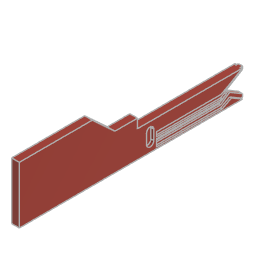
3ks (Autodesk Fusion 360 design; units mm, degrees)
Autodesk Fusion 360 part; units mm, degrees
note: some values were not read from the file. Set by a fixed rule: which face or edge a step refers to.
sketch "blade" plane through (0, 0, 0) normal (1, 0, 0) x (0, 1, 0)
  line L0 (0, 0) -> (0, 0.75) construction
  line L1 (0, 0.75) -> (25.25, 0.75)
  line L2 (25.25, 0.75) -> (25.25, 8.75)
  line L3 (25.25, 8.75) -> (0, 8.75)
  line L4 (0, 8.75) -> (0, 0.75)
  dimension "d14" = 0.75
  dimension "d15" = 25.25
  dimension "d16" = 8
  constraint coincident L0.start origin
  constraint vertical L0
  constraint horizontal L1
  constraint vertical L2
  constraint horizontal L3
  constraint vertical L4
  measures "d14" distance of L0.start L0.end
  measures "d15" distance of L0.end L1.end
  measures "d16" distance of L0.end L3.end
extrude "Extrude1" add sketch "blade" along normal blind 1.1 makes body 1
sketch "single track" plane through (1.1, 0, 0) normal (1, 0, 0) x (0, 1, 0)
  line L0 (0, 8.75) -> (0, 0.75)
  line L1 (0, 0.75) -> (25.25, 0.75)
  line L2 (25.25, 0.75) -> (25.25, 8.75)
  line L3 (25.25, 8.75) -> (0, 8.75)
  line L4 (0, 0.75) -> (0.9, 0.75) construction
  line L5 (0.9, 0.75) -> (4.4, 0.75) construction
  line L6 (4.4, 0.75) -> (7.9, 0.75) construction
  line L7 (7.9, 0.75) -> (11.4, 0.75) construction
  line L8 (11.4, 0.75) -> (14.9, 0.75) construction
  line L9 (14.9, 0.75) -> (18.4, 0.75) construction
  line L10 (0.9, 0.75) -> (0.9, 2.75) construction
  line L11 (4.4, 0.75) -> (4.4, 2.75) construction
  line L12 (7.9, 0.75) -> (7.9, 2.75) construction
  line L13 (11.4, 0.75) -> (11.4, 2.75) construction
  line L14 (14.9, 0.75) -> (14.9, 2.75) construction
  line L15 (18.4, 0.75) -> (18.4, 2.75) construction
  circle A0 centre (0.9, 2.75) radius 0.6375 construction
  circle A1 centre (4.4, 2.75) radius 0.6375 construction
  circle A2 centre (7.9, 2.75) radius 0.6375 construction
  circle A3 centre (11.4, 2.75) radius 0.6375 construction
  circle A4 centre (14.9, 2.75) radius 0.6375 construction
  circle A5 centre (18.4, 2.75) radius 0.6375 construction
  line L16 (0.9, 2.75) -> (0, 2.75)
  line L17 (0, 0.75) -> (0, 2.75) construction
  line L18 (0.9, 2.75) -> (1.2375, 2.75)
  line L19 (4.4, 2.75) -> (4.0625, 2.75)
  line L20 (4.4, 2.75) -> (4.7375, 2.75)
  line L21 (7.9, 2.75) -> (7.5625, 2.75)
  line L22 (7.9, 2.75) -> (8.2375, 2.75)
  line L23 (11.4, 2.75) -> (11.0625, 2.75)
  line L24 (11.4, 2.75) -> (11.7375, 2.75)
  line L25 (14.9, 2.75) -> (14.5625, 2.75)
  line L26 (14.9, 2.75) -> (15.2375, 2.75)
  line L27 (18.4, 2.75) -> (18.0625, 2.75)
  line L28 (18.4, 0.75) -> (21.9, 0.75) construction
  line L29 (18.4, 2.75) -> (18.7375, 2.75)
  line L30 (21.9, 0.75) -> (21.9, 4.75) construction
  line L31 (21.9, 4.75) -> (25.25, 4.75)
  line L32 (21.9, 4.75) -> (21.5625, 4.75)
  line L33 (1.2375, 2.75) -> (4.0625, 2.75)
  line L34 (4.7375, 2.75) -> (7.5625, 2.75)
  line L35 (8.2375, 2.75) -> (11.0625, 2.75)
  line L36 (11.7375, 2.75) -> (14.5625, 2.75)
  line L37 (15.2375, 2.75) -> (18.0625, 2.75)
  line L38 (18.7375, 2.75) -> (21.5625, 4.75)
  dimension "d19" = 0.9
  dimension "d20" = 3.5
  dimension "d21" = 3.5
  dimension "d22" = 3.5
  dimension "d23" = 3.5
  dimension "d24" = 3.5
  dimension "d25" = 2
  dimension "d26" = 2
  dimension "d27" = 2
  dimension "d28" = 2
  dimension "d29" = 2
  dimension "d30" = 2
  dimension "d31" = 1.275
  dimension "d32" = 1.275
  dimension "d33" = 1.275
  dimension "d34" = 1.275
  dimension "d35" = 1.275
  dimension "d36" = 1.275
  dimension "d37" = 0.3375
  dimension "d38" = 0.3375
  dimension "d39" = 0.3375
  dimension "d40" = 0.3375
  dimension "d41" = 0.3375
  dimension "d42" = 0.3375
  dimension "d43" = 0.3375
  dimension "d44" = 0.3375
  dimension "d45" = 0.3375
  dimension "d46" = 0.3375
  dimension "d47" = 3.5
  dimension "d48" = 0.3375
  dimension "d49" = 0.3375
  constraint coincident L0.end L1.start
  constraint perpendicular L0 L4
  constraint parallel L1 L5
  constraint parallel L1 L6
  constraint parallel L1 L7
  constraint parallel L1 L8
  constraint parallel L1 L9
  constraint perpendicular L5 L10
  constraint perpendicular L5 L11
  constraint perpendicular L7 L12
  constraint perpendicular L8 L13
  constraint perpendicular L1 L14
  constraint perpendicular L9 L15
  constraint coincident L10.end A0.centre
  constraint coincident L11.end A1.centre
  constraint coincident L12.end A2.centre
  constraint coincident L13.end A3.centre
  constraint coincident L14.end A4.centre
  constraint coincident L15.end A5.centre
  constraint coincident L0 L16.end
  constraint perpendicular L0 L16
  constraint perpendicular L10 L18
  constraint perpendicular L11 L19
  constraint perpendicular L11 L20
  constraint perpendicular L12 L21
  constraint perpendicular L12 L22
  constraint perpendicular L13 L23
  constraint perpendicular L13 L24
  constraint perpendicular L14 L25
  constraint perpendicular L14 L26
  constraint perpendicular L15 L27
  constraint perpendicular L15 L28
  constraint perpendicular L15 L29
  constraint perpendicular L28 L30
  constraint midpoint L2 L31.end
  constraint perpendicular L2 L31
  constraint perpendicular L30 L32
  measures "d19" distance of L0.end L4.end
  measures "d20" distance of L4.end L5.end
  measures "d21" distance of L5.end L6.end
  measures "d22" distance of L6.end L7.end
  measures "d23" distance of L7.end L8.end
  measures "d24" distance of L8.end L9.end
  measures "d25" distance of L4.end L10.end
  measures "d26" distance of L5.end L11.end
  measures "d27" distance of L6.end L12.end
  measures "d28" distance of L7.end L13.end
  measures "d29" distance of L8.end L14.end
  measures "d30" distance of L9.end L15.end
  measures "d31" diameter of A0
  measures "d32" diameter of A1
  measures "d33" diameter of A2
  measures "d34" diameter of A3
  measures "d35" diameter of A4
  measures "d36" diameter of A5
  measures "d37" distance of L10.end L18.end
  measures "d38" distance of L11.end L19.end
  measures "d39" distance of L11.end L20.end
  measures "d40" distance of L12.end L21.end
  measures "d41" distance of L12.end L22.end
  measures "d42" distance of L13.end L23.end
  measures "d43" distance of L13.end L24.end
  measures "d44" distance of L14.end L25.end
  measures "d45" distance of L14.end L26.end
  measures "d46" distance of L15.end L27.end
  measures "d47" distance of L9.end L28.end
  measures "d48" distance of L15.end L29.end
  measures "d49" distance of L30.end L32.end
sketch "single track cutter" plane through (0, 0, 0) normal (0, -1, 0) x (1, 0, 0)
  line L0 (0, 0.75) -> (1.1, 0.75)
  line L1 (1.1, 0.75) -> (1.1, 8.75)
  line L2 (1.1, 8.75) -> (0, 8.75)
  line L3 (0, 8.75) -> (0, 0.75)
  line L4 (1.1, 2.75) -> (1.1, 2.1125)
  line L5 (1.1, 2.75) -> (1.1, 3.3875)
  line L6 (1.1, 3.3875) -> (0.1, 3.3875)
  line L7 (0.1, 3.3875) -> (0.1, 2.1125)
  line L8 (0.1, 2.1125) -> (1.1, 2.1125)
  point P0 (1.1, 2.75)
  dimension "d50" = 0.6375
  dimension "d51" = 0.6375
  dimension "d52" = 1
  constraint vertical L4
  constraint coincident P0 L4.start
  constraint parallel L1 L5
  constraint perpendicular L5 L6
  constraint perpendicular L6 L7
  constraint perpendicular L4 L8
  measures "d50" distance of P0 L4.end
  measures "d51" distance of P0 L5.end
  measures "d52" distance of L5.end L6.end
sketch "double track" plane through (1.1, 0, 0) normal (1, 0, 0) x (0, 1, 0)
  line L0 (0, 8.75) -> (0, 0.75)
  line L1 (0, 0.75) -> (25.25, 0.75)
  line L2 (25.25, 0.75) -> (25.25, 8.75)
  line L3 (25.25, 8.75) -> (0, 8.75)
  line L4 (0, 0.75) -> (0.9, 0.75) construction
  line L5 (0.9, 0.75) -> (4.4, 0.75) construction
  line L6 (4.4, 0.75) -> (7.9, 0.75) construction
  line L7 (7.9, 0.75) -> (11.4, 0.75) construction
  line L8 (11.4, 0.75) -> (14.9, 0.75) construction
  line L9 (14.9, 0.75) -> (18.4, 0.75) construction
  line L10 (18.4, 0.75) -> (21.9, 0.75) construction
  line L11 (21.9, 0.75) -> (21.9, 4.75) construction
  line L12 (21.9, 4.75) -> (25.25, 4.75) construction
  line L13 (0.9, 0.75) -> (0.9, 3.25) construction
  line L14 (4.4, 0.75) -> (4.4, 3.25) construction
  line L15 (7.9, 0.75) -> (7.9, 3.25) construction
  line L16 (11.4, 0.75) -> (11.4, 3.25) construction
  line L17 (14.9, 0.75) -> (14.9, 3.25) construction
  line L18 (18.4, 0.75) -> (18.4, 3.25) construction
  line L19 (0.9, 3.25) -> (0.9, 2) construction
  line L20 (0.9, 3.25) -> (0.9, 4.5) construction
  line L21 (4.4, 3.25) -> (4.4, 2) construction
  line L22 (4.4, 3.25) -> (4.4, 4.5) construction
  line L23 (7.9, 3.25) -> (7.9, 2) construction
  line L24 (7.9, 3.25) -> (7.9, 4.5) construction
  line L25 (11.4, 3.25) -> (11.4, 2) construction
  line L26 (11.4, 3.25) -> (11.4, 4.5) construction
  line L27 (14.9, 3.25) -> (14.9, 2) construction
  line L28 (14.9, 3.25) -> (14.9, 4.5) construction
  line L29 (18.4, 3.25) -> (18.4, 2) construction
  line L30 (18.4, 3.25) -> (18.4, 4.5) construction
  line L31 (21.9, 4.75) -> (21.9, 3.5) construction
  line L32 (21.9, 4.75) -> (21.9, 6) construction
  circle A0 centre (0.9, 2) radius 0.6375 construction
  circle A1 centre (0.9, 4.5) radius 0.6375 construction
  circle A2 centre (4.4, 2) radius 0.6375 construction
  circle A3 centre (4.4, 4.5) radius 0.6375 construction
  circle A4 centre (7.9, 2) radius 0.6375 construction
  circle A5 centre (7.9, 4.5) radius 0.6375 construction
  circle A6 centre (11.4, 2) radius 0.6375 construction
  circle A7 centre (11.4, 4.5) radius 0.6375 construction
  circle A8 centre (14.9, 2) radius 0.6375 construction
  circle A9 centre (14.9, 4.5) radius 0.6375 construction
  circle A10 centre (18.4, 2) radius 0.6375 construction
  circle A11 centre (18.4, 4.5) radius 0.6375 construction
  line L33 (0.9, 2) -> (0, 2)
  line L34 (0.9, 4.5) -> (0, 4.5)
  line L35 (0, 0.75) -> (0, 2) construction
  line L36 (0, 0.75) -> (0, 4.5) construction
  line L37 (0.9, 2) -> (1.2375, 2)
  line L38 (4.4, 2) -> (4.0625, 2)
  line L39 (4.4, 2) -> (4.7375, 2)
  line L40 (7.9, 2) -> (7.5625, 2)
  line L41 (7.9, 2) -> (8.2375, 2)
  line L42 (11.4, 2) -> (11.0625, 2)
  line L43 (11.4, 2) -> (11.7375, 2)
  line L44 (14.9, 2) -> (14.5625, 2)
  line L45 (14.9, 2) -> (15.2375, 2)
  line L46 (18.4, 2) -> (18.0625, 2)
  line L47 (18.4, 2) -> (18.7375, 2)
  line L48 (21.9, 3.5) -> (21.5625, 3.5) construction
  line L49 (0.9, 4.5) -> (1.2375, 4.5)
  line L50 (4.4, 4.5) -> (4.0625, 4.5)
  line L51 (4.4, 4.5) -> (4.7375, 4.5)
  line L52 (7.9, 4.5) -> (7.5625, 4.5)
  line L53 (7.9, 4.5) -> (8.2375, 4.5)
  line L54 (11.4, 4.5) -> (11.0625, 4.5)
  line L55 (11.4, 4.5) -> (11.7375, 4.5)
  line L56 (14.9, 4.5) -> (14.5625, 4.5)
  line L57 (14.9, 4.5) -> (15.2375, 4.5)
  line L58 (18.4, 4.5) -> (18.0625, 4.5)
  line L59 (18.4, 4.5) -> (18.7375, 4.5)
  line L60 (21.9, 6) -> (21.5625, 6) construction
  line L61 (1.2375, 2) -> (4.0625, 2)
  line L62 (4.7375, 2) -> (7.5625, 2)
  line L63 (8.2375, 2) -> (11.0625, 2)
  line L64 (11.7375, 2) -> (14.5625, 2)
  line L65 (15.2375, 2) -> (18.0625, 2)
  line L66 (18.7375, 2) -> (21.5625, 3.5)
  line L67 (21.5625, 3.5) -> (25.25, 1.3192)
  line L68 (21.5625, 3.5) -> (25.25, 3.5) construction
  line L69 (25.25, 1.3192) -> (26.3259, 0.6829)
  line L70 (1.2375, 4.5) -> (4.0625, 4.5)
  line L71 (4.7375, 4.5) -> (7.5625, 4.5)
  line L72 (8.2375, 4.5) -> (11.0625, 4.5)
  line L73 (11.7375, 4.5) -> (14.5625, 4.5)
  line L74 (15.2375, 4.5) -> (18.0625, 4.5)
  line L75 (18.7375, 4.5) -> (21.5625, 6)
  line L76 (21.5625, 6) -> (25.25, 8.1808)
  line L77 (21.5625, 6) -> (25.25, 6) construction
  line L78 (25.25, 8.1808) -> (26.3259, 8.8171)
  dimension "d53" = 0.9
  dimension "d54" = 3.5
  dimension "d55" = 3.5
  dimension "d56" = 3.5
  dimension "d57" = 3.5
  dimension "d58" = 3.5
  dimension "d59" = 3.5
  dimension "d60" = 2.5
  dimension "d61" = 2.5
  dimension "d62" = 2.5
  dimension "d63" = 2.5
  dimension "d64" = 2.5
  dimension "d65" = 2.5
  dimension "d66" = 1.25
  dimension "d67" = 1.25
  dimension "d68" = 1.25
  dimension "d69" = 1.25
  dimension "d70" = 1.25
  dimension "d71" = 1.25
  dimension "d72" = 1.25
  dimension "d73" = 1.25
  dimension "d74" = 1.25
  dimension "d75" = 1.25
  dimension "d76" = 1.25
  dimension "d77" = 1.25
  dimension "d78" = 1.25
  dimension "d79" = 1.25
  dimension "d80" = 1.275
  dimension "d81" = 1.275
  dimension "d82" = 1.275
  dimension "d83" = 1.275
  dimension "d84" = 1.275
  dimension "d85" = 1.275
  dimension "d86" = 1.275
  dimension "d87" = 1.275
  dimension "d88" = 1.275
  dimension "d89" = 1.275
  dimension "d90" = 1.275
  dimension "d91" = 1.275
  dimension "d92" = 0.3375
  dimension "d93" = 0.3375
  dimension "d94" = 0.3375
  dimension "d95" = 0.3375
  dimension "d96" = 0.3375
  dimension "d97" = 0.3375
  dimension "d98" = 0.3375
  dimension "d99" = 0.3375
  dimension "d100" = 0.3375
  dimension "d101" = 0.3375
  dimension "d102" = 0.3375
  dimension "d103" = 0.3375
  dimension "d104" = 0.3375
  dimension "d105" = 0.3375
  dimension "d106" = 0.3375
  dimension "d107" = 0.3375
  dimension "d108" = 0.3375
  dimension "d109" = 0.3375
  dimension "d110" = 0.3375
  dimension "d111" = 0.3375
  dimension "d112" = 0.3375
  dimension "d113" = 0.3375
  dimension "d114" = 0.3375
  dimension "d115" = 0.3375
  dimension "d116" = 149.4
  dimension "d117" = 1.25
  dimension "d118" = 149.4
  dimension "d119" = 1.25
  constraint coincident L0.end L1.start
  constraint perpendicular L0 L4
  constraint parallel L1 L5
  constraint parallel L1 L6
  constraint parallel L1 L7
  constraint parallel L1 L8
  constraint parallel L1 L9
  constraint parallel L1 L10
  constraint perpendicular L10 L11
  constraint midpoint L2 L12.end
  constraint perpendicular L2 L12
  constraint perpendicular L5 L13
  constraint perpendicular L5 L14
  constraint perpendicular L7 L15
  constraint perpendicular L1 L16
  constraint perpendicular L8 L17
  constraint perpendicular L9 L18
  constraint parallel L13 L19
  constraint parallel L19 L20
  constraint parallel L14 L21
  constraint parallel L21 L22
  constraint parallel L15 L23
  constraint parallel L15 L24
  constraint parallel L16 L25
  constraint parallel L25 L26
  constraint parallel L17 L27
  constraint parallel L17 L28
  constraint parallel L18 L29
  constraint parallel L18 L30
  constraint perpendicular L12 L31
  constraint perpendicular L12 L32
  constraint coincident L19.end A0.centre
  constraint coincident L20.end A1.centre
  constraint coincident L21.end A2.centre
  constraint coincident L22.end A3.centre
  constraint coincident L23.end A4.centre
  constraint coincident L24.end A5.centre
  constraint coincident L25.end A6.centre
  constraint coincident L26.end A7.centre
  constraint coincident L27.end A8.centre
  constraint coincident L28.end A9.centre
  constraint coincident L29.end A10.centre
  constraint coincident L30.end A11.centre
  constraint coincident L0 L33.end
  constraint perpendicular L0 L33
  constraint coincident L0 L34.end
  constraint perpendicular L0 L34
  constraint perpendicular L13 L37
  constraint perpendicular L14 L38
  constraint perpendicular L21 L39
  constraint perpendicular L15 L40
  constraint perpendicular L15 L41
  constraint perpendicular L16 L42
  constraint perpendicular L16 L43
  constraint perpendicular L17 L44
  constraint perpendicular L17 L45
  constraint perpendicular L29 L46
  constraint perpendicular L29 L47
  constraint perpendicular L31 L48
  constraint perpendicular L20 L49
  constraint perpendicular L22 L50
  constraint perpendicular L22 L51
  constraint perpendicular L24 L52
  constraint perpendicular L24 L53
  constraint perpendicular L26 L54
  constraint perpendicular L26 L55
  constraint perpendicular L28 L56
  constraint perpendicular L28 L57
  constraint perpendicular L30 L58
  constraint perpendicular L30 L59
  constraint perpendicular L32 L60
  constraint horizontal L68
  constraint coincident L2 L67.end
  constraint coincident L2 L68.end
  constraint parallel L67 L69
  constraint horizontal L77
  constraint coincident L2 L76.end
  constraint coincident L2 L77.end
  constraint parallel L76 L78
  measures "d53" distance of L0.end L4.end
  measures "d54" distance of L4.end L5.end
  measures "d55" distance of L5.end L6.end
  measures "d56" distance of L6.end L7.end
  measures "d57" distance of L7.end L8.end
  measures "d58" distance of L8.end L9.end
  measures "d59" distance of L9.end L10.end
  measures "d60" distance of L4.end L13.end
  measures "d61" distance of L5.end L14.end
  measures "d62" distance of L6.end L15.end
  measures "d63" distance of L7.end L16.end
  measures "d64" distance of L8.end L17.end
  measures "d65" distance of L9.end L18.end
  measures "d66" distance of L13.end L19.end
  measures "d67" distance of L13.end L20.end
  measures "d68" distance of L14.end L21.end
  measures "d69" distance of L14.end L22.end
  measures "d70" distance of L15.end L23.end
  measures "d71" distance of L15.end L24.end
  measures "d72" distance of L16.end L25.end
  measures "d73" distance of L16.end L26.end
  measures "d74" distance of L17.end L27.end
  measures "d75" distance of L17.end L28.end
  measures "d76" distance of L18.end L29.end
  measures "d77" distance of L18.end L30.end
  measures "d78" distance of L11.end L31.end
  measures "d79" distance of L11.end L32.end
  measures "d80" diameter of A0
  measures "d81" diameter of A1
  measures "d82" diameter of A2
  measures "d83" diameter of A3
  measures "d84" diameter of A4
  measures "d85" diameter of A5
  measures "d86" diameter of A6
  measures "d87" diameter of A7
  measures "d88" diameter of A8
  measures "d89" diameter of A9
  measures "d90" diameter of A10
  measures "d91" diameter of A11
  measures "d92" distance of L19.end L37.end
  measures "d93" distance of L21.end L38.end
  measures "d94" distance of L21.end L39.end
  measures "d95" distance of L23.end L40.end
  measures "d96" distance of L23.end L41.end
  measures "d97" distance of L25.end L42.end
  measures "d98" distance of L25.end L43.end
  measures "d99" distance of L27.end L44.end
  measures "d100" distance of L27.end L45.end
  measures "d101" distance of L29.end L46.end
  measures "d102" distance of L29.end L47.end
  measures "d103" distance of L31.end L48.end
  measures "d104" distance of L20.end L49.end
  measures "d105" distance of L22.end L50.end
  measures "d106" distance of L22.end L51.end
  measures "d107" distance of L24.end L52.end
  measures "d108" distance of L24.end L53.end
  measures "d109" distance of L26.end L54.end
  measures "d110" distance of L26.end L55.end
  measures "d111" distance of L28.end L56.end
  measures "d112" distance of L28.end L57.end
  measures "d113" distance of L30.end L58.end
  measures "d114" distance of L30.end L59.end
  measures "d115" distance of L32.end L60.end
  measures "d116" angle of L67 L68
  measures "d117" distance of L67.end L69.end
  measures "d118" angle of L76 L77
  measures "d119" distance of L76.end L78.end
sketch "double track cutter" plane through (0, 0, 0) normal (0, -1, 0) x (1, 0, 0)
  line L0 (0, 0.75) -> (1.1, 0.75)
  line L1 (1.1, 0.75) -> (1.1, 8.75)
  line L2 (1.1, 8.75) -> (0, 8.75)
  line L3 (0, 8.75) -> (0, 0.75)
  line L4 (1.1, 2) -> (1.1, 1.3625)
  line L5 (1.1, 4.5) -> (1.1, 3.8625)
  line L6 (1.1, 2) -> (1.1, 2.6375)
  line L7 (1.1, 4.5) -> (1.1, 5.1375)
  line L8 (1.1, 1.3625) -> (0.6, 1.3625)
  line L9 (1.1, 3.8625) -> (0.6, 3.8625)
  line L10 (0.6, 1.3625) -> (0.6, 2.6375)
  line L11 (0.6, 2.6375) -> (1.1, 2.6375)
  line L12 (0.6, 3.8625) -> (0.6, 5.1375)
  line L13 (0.6, 5.1375) -> (1.1, 5.1375)
  point P0 (1.1, 2)
  point P1 (1.1, 4.5)
  dimension "d120" = 0.6375
  dimension "d121" = 0.6375
  dimension "d122" = 0.6375
  dimension "d123" = 0.6375
  dimension "d124" = 0.5
  dimension "d125" = 0.5
  constraint vertical L4
  constraint coincident P0 L4.start
  constraint vertical L5
  constraint coincident P1 L5.start
  constraint parallel L1 L6
  constraint parallel L1 L7
  constraint perpendicular L4 L8
  constraint perpendicular L5 L9
  constraint perpendicular L8 L10
  constraint perpendicular L6 L11
  constraint perpendicular L9 L12
  constraint perpendicular L7 L13
  measures "d120" distance of P0 L4.end
  measures "d121" distance of P1 L5.end
  measures "d122" distance of P0 L6.end
  measures "d123" distance of P1 L7.end
  measures "d124" distance of L4.end L8.end
  measures "d125" distance of L5.end L9.end
extrude "sidebar hole extension" add 1 faces at (0.3667, 0, 6.0833) along direction (0, -1, 0) blind 5.5 on bodies 1 bodies 1
sketch "sidebar hole" plane through (1.1, 0, 0) normal (1, 0, 0) x (0, 1, 0)
  line L0 (-5.5, 0.75) -> (25.25, 0.75)
  line L1 (25.25, 0.75) -> (25.25, 8.75)
  line L2 (25.25, 8.75) -> (-5.5, 8.75)
  line L3 (-5.5, 8.75) -> (-5.5, 0.75)
  line L4 (-5.5, 0.75) -> (0, 0.75) construction
  line L5 (0, 0.75) -> (0, 4.75) construction
  line L6 (0, 4.75) -> (-2.9, 4.75) construction
  line L7 (-2.9, 4.75) -> (-2.9, 3.3)
  line L8 (-2.9, 3.3) -> (-2.9, 2.25) construction
  line L9 (-2.9, 2.25) -> (-0.8, 2.25) construction
  line L10 (-0.8, 2.25) -> (-0.8, 3.3) construction
  line L11 (-2.9, 4.75) -> (-2.9, 6.2)
  line L12 (-2.9, 6.2) -> (-2.9, 7.25) construction
  line L13 (-2.9, 7.25) -> (-0.8, 7.25) construction
  line L14 (-0.8, 7.25) -> (-0.8, 6.2) construction
  line L15 (-0.8, 6.2) -> (-0.8, 3.3)
  arc A0 (-2.9, 3.3) -> (-0.8, 3.3) centre (-1.85, 3.3) ccw
  arc A1 (-0.8, 6.2) -> (-2.9, 6.2) centre (-1.85, 6.2) ccw
  dimension "d128" = 5.5
  dimension "d129" = 4
  dimension "d130" = 2.9
  dimension "d131" = 1.45
  dimension "d132" = 1.05
  dimension "d133" = 2.1
  dimension "d134" = 1.05
  dimension "d135" = 1.45
  dimension "d136" = 1.05
  dimension "d137" = 2.1
  dimension "d138" = 1.05
  constraint coincident L0.start L3.end
  constraint perpendicular L3 L4
  constraint perpendicular L4 L5
  constraint perpendicular L5 L6
  constraint perpendicular L6 L7
  constraint parallel L7 L8
  constraint perpendicular L8 L9
  constraint perpendicular L9 L10
  constraint perpendicular L6 L11
  constraint parallel L11 L12
  constraint perpendicular L12 L13
  constraint perpendicular L13 L14
  constraint tangent L9 A0
  constraint tangent L13 A1
  measures "d128" distance of L0.start L4.end
  measures "d129" distance of L4.end L5.end
  measures "d130" distance of L5.end L6.end
  measures "d131" distance of L6.end L7.end
  measures "d132" distance of L7.end L8.end
  measures "d133" distance of L8.end L9.end
  measures "d134" distance of L9.end L10.end
  measures "d135" distance of L6.end L11.end
  measures "d136" distance of L11.end L12.end
  measures "d137" distance of L12.end L13.end
  measures "d138" distance of L13.end L14.end
sketch "feed ramp" plane through (1.1, 0, 0) normal (1, 0, 0) x (0, 1, 0)
  line L0 (-5.5, 0.75) -> (25.25, 0.75)
  line L1 (25.25, 0.75) -> (25.25, 8.75)
  line L2 (25.25, 8.75) -> (-5.5, 8.75)
  line L3 (-5.5, 8.75) -> (-5.5, 0.75)
  line L4 (25.25, 0.75) -> (25.25, 4.75) construction
  line L5 (25.25, 4.75) -> (21.9, 4.75) construction
  line L6 (21.9, 4.75) -> (21.9, 6) construction
  line L7 (21.9, 4.75) -> (21.9, 3.5) construction
  line L8 (21.9, 6) -> (22.2375, 6) construction
  line L9 (21.9, 3.5) -> (22.2375, 3.5) construction
  line L10 (22.2375, 6) -> (25.25, 7.7816)
  line L11 (22.2375, 6) -> (25.25, 6) construction
  line L12 (22.2375, 3.5) -> (25.25, 1.7184)
  line L13 (22.2375, 3.5) -> (25.25, 3.5) construction
  line L14 (22.2375, 6) -> (20.1239, 4.75)
  line L15 (22.2375, 3.5) -> (20.1239, 4.75)
  dimension "d139" = 3.35
  dimension "d140" = 1.25
  dimension "d141" = 1.25
  dimension "d142" = 0.3375
  dimension "d143" = 0.3375
  dimension "d144" = 149.4
  dimension "d145" = 149.4
  constraint coincident L0.end L1.start
  constraint midpoint L1 L4.end
  constraint perpendicular L4 L5
  constraint perpendicular L5 L6
  constraint perpendicular L5 L7
  constraint perpendicular L6 L8
  constraint perpendicular L7 L9
  constraint horizontal L11
  constraint coincident L1 L10.end
  constraint coincident L1 L11.end
  constraint horizontal L13
  constraint coincident L4 L12.end
  constraint coincident L4 L13.end
  constraint parallel L10 L14
  constraint coincident L14 L15.end
  constraint parallel L12 L15
  constraint coincident L14.end L15.end
  measures "d139" distance of L4.end L5.end
  measures "d140" distance of L5.end L6.end
  measures "d141" distance of L5.end L7.end
  measures "d142" distance of L6.end L8.end
  measures "d143" distance of L7.end L9.end
  measures "d144" angle of L10 L11
  measures "d145" angle of L12 L13
sketch "bow" plane through (1.1, 0, 0) normal (1, 0, 0) x (0, 1, 0)
  line L0 (-5.5, 0.75) -> (25.25, 0.75)
  line L1 (25.25, 0.75) -> (25.25, 8.75)
  line L2 (25.25, 8.75) -> (-5.5, 8.75)
  line L3 (-5.5, 8.75) -> (-5.5, 0.75)
  line L4 (-5.5, 0.75) -> (-39.5, 0.75)
  line L5 (-39.5, 0.75) -> (-39.5, 17.25)
  line L6 (-39.5, 17.25) -> (-18.5, 17.25)
  line L7 (-5.5, 8.75) -> (-5.5, 11.25)
  line L8 (-5.5, 11.25) -> (-12, 11.25)
  line L9 (-12, 11.25) -> (-18.5, 17.25)
  dimension "d146" = 34
  dimension "d147" = 16.5
  dimension "d148" = 21
  dimension "d149" = 2.5
  dimension "d150" = 6.5
  constraint coincident L0.start L3.end
  constraint perpendicular L3 L4
  constraint perpendicular L4 L5
  constraint perpendicular L5 L6
  constraint coincident L2.end L3.start
  constraint perpendicular L2 L7
  constraint perpendicular L7 L8
  measures "d146" distance of L0.start L4.end
  measures "d147" distance of L4.end L5.end
  measures "d148" distance of L5.end L6.end
  measures "d149" distance of L2.end L7.end
  measures "d150" distance of L7.end L8.end
extrude "Extrude3" cut sketch "sidebar hole" against normal blind 0.85 contours L7 L11 L15 A0 A1 bodies 1
extrude "Extrude4" cut sketch "feed ramp" against normal blind 1.1 contours L1 L10 L12 L14 L15 bodies 1
sweep "Sweep1" cut profiles "single track cutter" path "single track" along L31 L32 L38 L29 L27 L37 L26 L25 L36 L24 L23 L35 L22 L21 L34 L20 L19 L33 L18 L16 section 1 contours L1 L4 L5 L6 L7 L8 bodies 1
sweep "Sweep2" cut profiles "double track cutter" path "double track" along L33 L37 L61 L38 L39 L62 L40 L41 L63 L42 L43 L64 L44 L45 L65 L46 L47 L66 L67 L69 section 1 contours L1 L4 L6 L8 L10 L11 bodies 1
sweep "Sweep3" cut profiles "double track cutter" path "double track" along L78 L76 L75 L59 L58 L74 L57 L56 L73 L55 L54 L72 L53 L52 L71 L51 L50 L70 L49 L34 section 1 contours L1 L5 L7 L9 L12 L13 bodies 1
copy_body "CopyPasteBodies1" bodies 1 makes body 2
move_body "Move1" bodies 2 to x (-1, 0, 0) y (0, 1, 0) z (0, 0, -1) at (0, 0, 1.5)
move_body "Move2" bodies 2 to x (1, 0, 0) y (0, 1, 0) z (0, 0, 1) at (0, 0, 8)
extrude "Extrude5" add sketch "bow" against normal blind 2.2 contours L3 L4 L5 L6 L7 L8 L9 bodies 1 2
move_face "OffsetFaces1" offset -0.125 2 faces at (-0.2, 4.6534, 8.75) (0.2, -18.0133, 0.75) on bodies 1
equation "Single1 = 1 mm"
equation "Single2 = 1 mm"
equation "Single3 = 1 mm"
equation "Single4 = 1 mm"
equation "Single5 = 1 mm"
equation "Single6 = 1 mm"
equation "Double1 = 1 mm"
equation "Double2 = 1 mm"
equation "Double3 = 1 mm"
equation "Double4 = 1 mm"
equation "Double5 = 1 mm"
equation "Double6 = 1 mm"
equation "TrackToleranceAdd = 0.075 mm"
equation "d21 = d20"
equation "d22 = d20"
equation "d23 = d20"
equation "d24 = d20"
equation "d25 = 1.5 mm + 0.5 * Single1"
equation "d26 = 1.5 mm + 0.5 * Single2"
equation "d27 = 1.5 mm + 0.5 * Single3"
equation "d28 = 1.5 mm + 0.5 * Single4"
equation "d29 = 1.5 mm + 0.5 * Single5"
equation "d30 = 1.5 mm + 0.5 * Single6"
equation "d31 = 1.2 mm + TrackToleranceAdd"
equation "d32 = d31"
equation "d33 = d31"
equation "d34 = d31"
equation "d35 = d31"
equation "d36 = d31"
equation "d37 = 0.3 mm + 0.5 * TrackToleranceAdd"
equation "d38 = d37"
equation "d39 = d37"
equation "d40 = d37"
equation "d41 = d37"
equation "d42 = d37"
equation "d43 = d37"
equation "d44 = d37"
equation "d45 = d37"
equation "d46 = d37"
equation "d47 = d20"
equation "d48 = d37"
equation "d49 = d37"
equation "d50 = 0.5 * d31"
equation "d51 = d50"
equation "d53 = d19"
equation "d54 = d20"
equation "d55 = d20"
equation "d56 = d20"
equation "d57 = d20"
equation "d58 = d20"
equation "d59 = d20"
equation "d60 = 2 mm + 0.5 * Double1"
equation "d61 = 2 mm + 0.5 * Double2"
equation "d62 = 2 mm + 0.5 * Double3"
equation "d63 = 2 mm + 0.5 * Double4"
equation "d64 = 2 mm + 0.5 * Double5"
equation "d65 = 2 mm + 0.5 * Double6"
equation "d67 = d66"
equation "d68 = d66"
equation "d69 = d66"
equation "d70 = d66"
equation "d71 = d66"
equation "d72 = d66"
equation "d73 = d66"
equation "d74 = d66"
equation "d75 = d66"
equation "d76 = d66"
equation "d77 = d66"
equation "d78 = d66"
equation "d79 = d66"
equation "d80 = d31"
equation "d81 = d31"
equation "d82 = d31"
equation "d83 = d31"
equation "d84 = d31"
equation "d85 = d31"
equation "d86 = d31"
equation "d87 = d31"
equation "d88 = d31"
equation "d89 = d31"
equation "d90 = d31"
equation "d91 = d31"
equation "d92 = d37"
equation "d93 = d37"
equation "d94 = d37"
equation "d95 = d37"
equation "d96 = d37"
equation "d97 = d37"
equation "d98 = d37"
equation "d99 = d37"
equation "d100 = d37"
equation "d101 = d37"
equation "d102 = d37"
equation "d103 = d37"
equation "d104 = d37"
equation "d105 = d37"
equation "d106 = d37"
equation "d107 = d37"
equation "d108 = d37"
equation "d109 = d37"
equation "d110 = d37"
equation "d111 = d37"
equation "d112 = d37"
equation "d113 = d37"
equation "d114 = d37"
equation "d115 = d37"
equation "d117 = d66"
equation "d118 = d116"
equation "d119 = d66"
equation "d120 = d50"
equation "d121 = d50"
equation "d122 = d50"
equation "d123 = d50"
equation "d124 = 0.5 * d52"
equation "d125 = d124"
equation "d132 = 2.5 mm - d131"
equation "d134 = d132"
equation "d135 = d131"
equation "d136 = d132"
equation "d137 = d133"
equation "d138 = d132"
equation "d140 = d66"
equation "d141 = d66"
equation "d142 = d37"
equation "d143 = d37"
equation "d144 = d116"
equation "d145 = d116"
named bodies: "blade", "blade (1)"
